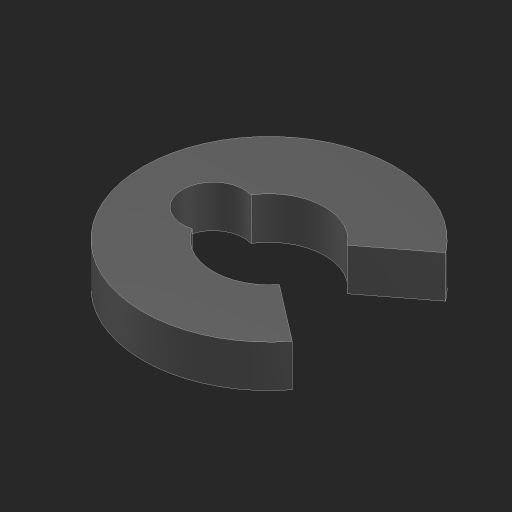
# Autodesk Inventor part: Spacer Nylon Click On
Saved by Autodesk Inventor 2023 (Build 270158000, 158)
## iProperties
Created: 2022-08-02
Part Number: Spacer Nylon Click On
Material: Generic
Document SubType Name: Modeling
Designer: ylu12
Density: 1 g/cm^3
Appearance: Black Nylon
Author: ylu12
Autodesk Inventor part; units mm, degrees
ref_plane "YZ Plane" through (0, 0, 0) normal (1, 0, 0) x (0, 1, 0)
ref_plane "XZ Plane" through (0, 0, 0) normal (0, 1, 0) x (-1, 0, 0)
ref_plane "XY Plane" through (0, 0, 0) normal (0, 0, 1) x (1, 0, 0)
sketch "Sketch1" plane through (0, 0, 0) normal (0, 1, 0) x (-1, 0, 0)
  circle A0 centre (0, 0) radius 4.7625
  circle A1 centre (0, 0) radius 2.1082
  circle A2 centre (2.1082, 0) radius 1.1557
  line L0 (-1.6725, 1.2834) -> (-3.7783, 2.8992)
  line L1 (-1.6725, -1.2834) -> (-3.7783, -2.8992)
  line L2 (2.1082, 0) -> (-4.7625, 0) construction
  point P0 (1.7914, 1.1114)
  point P1 (1.7914, -1.1114)
  dimension "d0" = 9.525
  dimension "d1" = 4.2164
  dimension "d2" = 2.3114
  dimension "d3" = 75
  constraints: 6 end point, 6 point on circle, 3 centre point, 2 coincident, 2 line through centre, 1 horizontal, 1 point on line, 1 other
  measures "d0" diameter of A0
  measures "d1" diameter of A1
  measures "d2" diameter of A2
  measures "d3" angle of L1 L0
extrude "Extrusion1" add sketch "Sketch1" along normal blind 1.5875 contours A0 L1 A1 A2 L0
body "Solid1"
